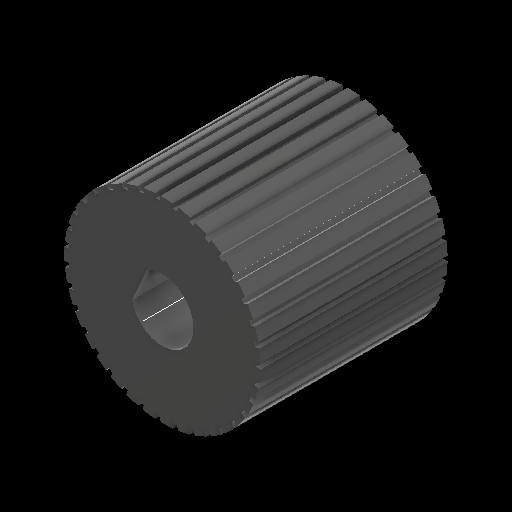
# Autodesk Inventor part: RobotWheelMK1printtest
Saved by Autodesk Inventor 2025 (Build 290162000, 162)
## iProperties
Created: 2024-11-18
Part Number: RobotWheelMK1printtest
Material: Generic
Document SubType Name: Modeling
Designer: Trevor
Density: 1 g/cm^3
Appearance: Default
Author: Trevor
Autodesk Inventor part; units mm, degrees
ref_plane "YZ Plane" through (0, 0, 0) normal (1, 0, 0) x (0, 1, 0)
ref_plane "XZ Plane" through (0, 0, 0) normal (0, 1, 0) x (-1, 0, 0)
ref_plane "XY Plane" through (0, 0, 0) normal (0, 0, 1) x (1, 0, 0)
sketch "Sketch1" plane through (0, 0, 0) normal (0, 0, 1) x (1, 0, 0)
  line L0 (-2.4408, -0.5408) -> (-1.2026, 2.1918) projected
  arc A0 (-2.4408, -0.5408) -> (-1.2026, 2.1918) centre (0, 0) ccw projected
  circle A1 centre (0, 0) radius 7.5
  line L1 (-7.8445, -0.4921) -> (-7.4838, -0.4921)
  line L2 (-7.4838, 0.4921) -> (-7.8445, 0.4921)
  line L3 (-7.8445, 0.4921) -> (-7.8445, -0.4921)
  line L4 (-7.8445, -0.4921) -> (-7.5, 0) construction
  line L5 (-7.5, 0) -> (-7.8445, 0.4921) construction
  line L6 (-7.4514, -0.8521) -> (-7.8063, -0.9165)
  line L7 (-7.8063, -0.9165) -> (-7.6306, -1.8849)
  line L8 (-7.6306, -1.8849) -> (-7.2757, -1.8205)
  circle A2 centre (0, 0) radius 7.5
  line L9 (-7.1795, -2.1689) -> (-7.5172, -2.2956)
  line L10 (-7.5172, -2.2956) -> (-7.1714, -3.2171)
  line L11 (-7.1714, -3.2171) -> (-6.8337, -3.0904)
  circle A3 centre (0, 0) radius 7.5
  line L12 (-6.6769, -3.416) -> (-6.9865, -3.601)
  line L13 (-6.9865, -3.601) -> (-6.4817, -4.4459)
  line L14 (-6.4817, -4.4459) -> (-6.1721, -4.2609)
  circle A4 centre (0, 0) radius 7.5
  line L15 (-5.9597, -4.5533) -> (-6.2312, -4.7906)
  line L16 (-6.2312, -4.7906) -> (-5.5837, -5.5318)
  line L17 (-5.5837, -5.5318) -> (-5.3121, -5.2945)
  circle A5 centre (0, 0) radius 7.5
  line L18 (-5.0509, -5.5443) -> (-5.2757, -5.8262)
  line L19 (-5.2757, -5.8262) -> (-4.5062, -6.4399)
  line L20 (-4.5062, -6.4399) -> (-4.2813, -6.1579)
  circle A6 centre (0, 0) radius 7.5
  line L21 (-3.9797, -6.357) -> (-4.1506, -6.6746)
  line L22 (-4.1506, -6.6746) -> (-3.2839, -7.141)
  line L23 (-3.2839, -7.141) -> (-3.113, -6.8234)
  circle A7 centre (0, 0) radius 7.5
  line L24 (-2.7807, -6.9655) -> (-2.8921, -7.3085)
  line L25 (-2.8921, -7.3085) -> (-1.956, -7.6126)
  line L26 (-1.956, -7.6126) -> (-1.8446, -7.2696)
  circle A8 centre (0, 0) radius 7.5
  line L27 (-1.4923, -7.35) -> (-1.5407, -7.7074)
  line L28 (-1.5407, -7.7074) -> (-0.5653, -7.8396)
  line L29 (-0.5653, -7.8396) -> (-0.5169, -7.4822)
  circle A9 centre (0, 0) radius 7.5
  line L30 (-0.1559, -7.4984) -> (-0.1397, -7.8587)
  line L31 (-0.1397, -7.8587) -> (0.8436, -7.8145)
  line L32 (0.8436, -7.8145) -> (0.8274, -7.4542)
  circle A10 centre (0, 0) radius 7.5
  line L33 (1.1855, -7.4057) -> (1.2658, -7.7573)
  line L34 (1.2658, -7.7573) -> (2.2254, -7.5383)
  line L35 (2.2254, -7.5383) -> (2.1451, -7.1867)
  circle A11 centre (0, 0) radius 7.5
  line L36 (2.4888, -7.075) -> (2.6306, -7.4066)
  line L37 (2.6306, -7.4066) -> (3.5356, -7.0198)
  line L38 (3.5356, -7.0198) -> (3.3939, -6.6882)
  circle A12 centre (0, 0) radius 7.5
  line L39 (3.7121, -6.5169) -> (3.9108, -6.8179)
  line L40 (3.9108, -6.8179) -> (4.7322, -6.2757)
  line L41 (4.7322, -6.2757) -> (4.5335, -5.9747)
  circle A13 centre (0, 0) radius 7.5
  line L42 (4.8161, -5.7494) -> (5.0653, -6.01)
  line L43 (5.0653, -6.01) -> (5.7767, -5.3299)
  line L44 (5.7767, -5.3299) -> (5.5275, -5.0692)
  circle A14 centre (0, 0) radius 7.5
  line L45 (5.7653, -4.797) -> (6.0571, -5.009)
  line L46 (6.0571, -5.009) -> (6.6356, -4.2127)
  line L47 (6.6356, -4.2127) -> (6.3438, -4.0008)
  circle A15 centre (0, 0) radius 7.5
  line L48 (6.5292, -3.6905) -> (6.8541, -3.847)
  line L49 (6.8541, -3.847) -> (7.2812, -2.9602)
  line L50 (7.2812, -2.9602) -> (6.9562, -2.8037)
  circle A16 centre (0, 0) radius 7.5
  line L51 (7.0832, -2.4654) -> (7.4309, -2.5613)
  line L52 (7.4309, -2.5613) -> (7.6927, -1.6125)
  line L53 (7.6927, -1.6125) -> (7.3451, -1.5166)
  circle A17 centre (0, 0) radius 7.5
  line L54 (7.4096, -1.161) -> (7.7688, -1.1933)
  line L55 (7.7688, -1.1933) -> (7.857, -0.213)
  line L56 (7.857, -0.213) -> (7.4978, -0.1807)
  circle A18 centre (0, 0) radius 7.5
  line L57 (7.4978, 0.1807) -> (7.857, 0.213)
  line L58 (7.857, 0.213) -> (7.7688, 1.1933)
  line L59 (7.7688, 1.1933) -> (7.4096, 1.161)
  circle A19 centre (0, 0) radius 7.5
  line L60 (7.3451, 1.5166) -> (7.6927, 1.6125)
  line L61 (7.6927, 1.6125) -> (7.4309, 2.5613)
  line L62 (7.4309, 2.5613) -> (7.0832, 2.4654)
  circle A20 centre (0, 0) radius 7.5
  line L63 (6.9562, 2.8037) -> (7.2812, 2.9602)
  line L64 (7.2812, 2.9602) -> (6.8541, 3.847)
  line L65 (6.8541, 3.847) -> (6.5292, 3.6905)
  circle A21 centre (0, 0) radius 7.5
  line L66 (6.3438, 4.0008) -> (6.6356, 4.2127)
  line L67 (6.6356, 4.2127) -> (6.0571, 5.009)
  line L68 (6.0571, 5.009) -> (5.7653, 4.797)
  circle A22 centre (0, 0) radius 7.5
  line L69 (5.5275, 5.0692) -> (5.7767, 5.3299)
  line L70 (5.7767, 5.3299) -> (5.0653, 6.01)
  line L71 (5.0653, 6.01) -> (4.8161, 5.7494)
  circle A23 centre (0, 0) radius 7.5
  line L72 (4.5335, 5.9747) -> (4.7322, 6.2757)
  line L73 (4.7322, 6.2757) -> (3.9108, 6.8179)
  line L74 (3.9108, 6.8179) -> (3.7121, 6.5169)
  circle A24 centre (0, 0) radius 7.5
  line L75 (3.3939, 6.6882) -> (3.5356, 7.0198)
  line L76 (3.5356, 7.0198) -> (2.6306, 7.4066)
  line L77 (2.6306, 7.4066) -> (2.4888, 7.075)
  circle A25 centre (0, 0) radius 7.5
  line L78 (2.1451, 7.1867) -> (2.2254, 7.5383)
  line L79 (2.2254, 7.5383) -> (1.2658, 7.7573)
  line L80 (1.2658, 7.7573) -> (1.1855, 7.4057)
  circle A26 centre (0, 0) radius 7.5
  line L81 (0.8274, 7.4542) -> (0.8436, 7.8145)
  line L82 (0.8436, 7.8145) -> (-0.1397, 7.8587)
  line L83 (-0.1397, 7.8587) -> (-0.1559, 7.4984)
  circle A27 centre (0, 0) radius 7.5
  line L84 (-0.5169, 7.4822) -> (-0.5653, 7.8396)
  line L85 (-0.5653, 7.8396) -> (-1.5407, 7.7074)
  line L86 (-1.5407, 7.7074) -> (-1.4923, 7.35)
  circle A28 centre (0, 0) radius 7.5
  line L87 (-1.8446, 7.2696) -> (-1.956, 7.6126)
  line L88 (-1.956, 7.6126) -> (-2.8921, 7.3085)
  line L89 (-2.8921, 7.3085) -> (-2.7807, 6.9655)
  circle A29 centre (0, 0) radius 7.5
  line L90 (-3.113, 6.8234) -> (-3.2839, 7.141)
  line L91 (-3.2839, 7.141) -> (-4.1506, 6.6746)
  line L92 (-4.1506, 6.6746) -> (-3.9797, 6.357)
  circle A30 centre (0, 0) radius 7.5
  line L93 (-4.2813, 6.1579) -> (-4.5062, 6.4399)
  line L94 (-4.5062, 6.4399) -> (-5.2757, 5.8262)
  line L95 (-5.2757, 5.8262) -> (-5.0509, 5.5443)
  circle A31 centre (0, 0) radius 7.5
  line L96 (-5.3121, 5.2945) -> (-5.5837, 5.5318)
  line L97 (-5.5837, 5.5318) -> (-6.2312, 4.7906)
  line L98 (-6.2312, 4.7906) -> (-5.9597, 4.5533)
  circle A32 centre (0, 0) radius 7.5
  line L99 (-6.1721, 4.2609) -> (-6.4817, 4.4459)
  line L100 (-6.4817, 4.4459) -> (-6.9865, 3.601)
  line L101 (-6.9865, 3.601) -> (-6.6769, 3.416)
  circle A33 centre (0, 0) radius 7.5
  line L102 (-6.8337, 3.0904) -> (-7.1714, 3.2171)
  line L103 (-7.1714, 3.2171) -> (-7.5172, 2.2956)
  line L104 (-7.5172, 2.2956) -> (-7.1795, 2.1689)
  circle A34 centre (0, 0) radius 7.5
  line L105 (-7.2757, 1.8205) -> (-7.6306, 1.8849)
  line L106 (-7.6306, 1.8849) -> (-7.8063, 0.9165)
  line L107 (-7.8063, 0.9165) -> (-7.4514, 0.8521)
  circle A35 centre (0, 0) radius 7.5
  point P0 (0, 0)
  point P1 (-7.3795, -1.3392)
  point P2 (-7.0218, -2.6353)
  point P3 (-6.4384, -3.8467)
  point P4 (-5.648, -4.9345)
  point P5 (-4.6762, -5.8637)
  point P6 (-3.554, -6.6045)
  point P7 (-2.3176, -7.1329)
  point P8 (-1.0067, -7.4321)
  point P9 (0.3365, -7.4924)
  point P10 (1.6689, -7.312)
  point P11 (2.9477, -6.8965)
  point P12 (4.1317, -6.2593)
  point P13 (5.183, -5.421)
  point P14 (6.0676, -4.4084)
  point P15 (6.7573, -3.2541)
  point P16 (7.2297, -1.9953)
  point P17 (7.4698, -0.6723)
  point P18 (7.4698, 0.6723)
  point P19 (7.2297, 1.9953)
  point P20 (6.7573, 3.2541)
  point P21 (6.0676, 4.4084)
  point P22 (5.183, 5.421)
  point P23 (4.1317, 6.2593)
  point P24 (2.9477, 6.8965)
  point P25 (1.6689, 7.312)
  point P26 (0.3365, 7.4924)
  point P27 (-1.0067, 7.4321)
  point P28 (-2.3176, 7.1329)
  point P29 (-3.554, 6.6045)
  point P30 (-4.6762, 5.8637)
  point P31 (-5.648, 4.9345)
  point P32 (-6.4384, 3.8467)
  point P33 (-7.0218, 2.6353)
  point P34 (-7.3795, 1.3392)
  dimension "d0" = 15
  dimension "d5" = 360
  constraints: 214 end point, 102 point on circle, 34 centre point, 2 coincident with centre, 1 coincident, 1 horizontal, 1 parallel, 354 other
ref_plane "Work Plane1" through (-2, -2, 15) normal (0, 0, 1) x (1, 0, 0)
extrude "Extrusion1" add sketch "Sketch1" along normal up to surface (15 mm away)
body "Solid1"
